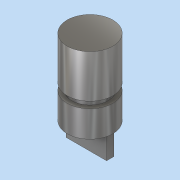
# Autodesk Inventor part: 00_IR_Laserdiode
Saved by Autodesk Inventor 2019.4 (Build 234330000, 330)
## iProperties
Created: 2020-11-30
Part Number: 00_IR_Laserdiode
Material: Generic
Document SubType Name: Modeling
Designer: diederichbenedict
Density: 1 g/cm^3
Appearance: Chrome - Polished
Author: diederichbenedict
Autodesk Inventor part; units mm, degrees
ref_plane "YZ Plane" through (0, 0, 0) normal (1, 0, 0) x (0, 1, 0)
ref_plane "XZ Plane" through (0, 0, 0) normal (0, 1, 0) x (-1, 0, 0)
ref_plane "XY Plane" through (0, 0, 0) normal (0, 0, 1) x (1, 0, 0)
sketch "Sketch1" plane through (0, 0, 0) normal (1, 0, 0) x (0, 1, 0)
  line L0 (0, 0) -> (6.52, 0)
  line L1 (6.52, 0) -> (6.52, -3)
  line L2 (6.52, -3) -> (0.86, -3)
  line L3 (0.86, -3) -> (0.86, -2.41)
  line L4 (0.86, -2.41) -> (0, -2.41)
  line L5 (0, -2.41) -> (0, 0)
  line L6 (0, -6.589) -> (-0.9134, -6.589)
  line L7 (0, 0) -> (-3.48, 0)
  line L8 (-3.48, 0) -> (-3.48, -3)
  line L9 (-3.48, -3) -> (0, -3)
  line L10 (0, -3) -> (0, 0)
  point P0 (-0.9134, 0)
  dimension "d1" = 3
  dimension "d2" = 5.66
  dimension "d6" = 0.86
  dimension "d8" = 10
  dimension "d9" = 2.41
  constraints: 22 end point, 6 perpendicular, 3 horizontal, 2 parallel, 2 point on line
  measures "d1" distance of L0.end L1.end
  measures "d2" distance of L1.end L2.end
  measures "d6" distance between parallel lines of L5 L3
  measures "d8" distance between parallel lines of L8 L1
  measures "d9" distance between parallel lines of L4 L0
revolve "Revolution1" add sketch "Sketch1" angle 360 about axis through (0, 0, 0) along (0, 1, 0)
sketch "Sketch2" plane through (0, -3.48, 0) normal (0, -1, 0) x (1, 0, 0)
  circle A0 centre (0, 0) radius 3 projected
  line L0 (2.673, -0.4849) -> (-2.673, -0.4849)
  line L1 (-2.673, -0.4849) -> (-2.673, 0.4849)
  line L2 (-2.673, 0.4849) -> (2.673, 0.4849)
  line L3 (2.673, 0.4849) -> (2.673, -0.4849)
  line L4 (2.673, -0.4849) -> (-2.673, 0.4849) construction
  line L5 (-2.673, -0.4849) -> (2.673, 0.4849) construction
  constraints: 12 end point, 2 midpoint, 2 parallel, 1 horizontal, 1 perpendicular
extrude "Extrusion1" add sketch "Sketch2" along normal blind 3 contours L0 L1 L2 L3
body "Solid1"
